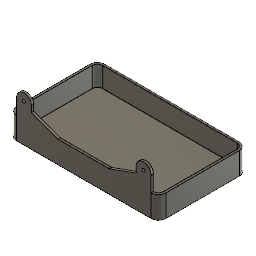
eka v1 v1 (Autodesk Fusion 360 design; units mm, degrees)
Autodesk Fusion 360 part; units mm, degrees
sketch "Sketch1" plane through (0, 0, 0) normal (0, 1, 0) x (1, 0, 0)
  line L0 (-190, 118.3432) -> (-10, 118.3432)
  line L1 (0, 108.3432) -> (0, 10)
  line L2 (-10, 0) -> (-190, 0)
  line L3 (-200, 10) -> (-200, 108.3432)
  arc A0 (-190, 118.3432) -> (-200, 108.3432) centre (-190, 108.3432) ccw
  arc A1 (-200, 10) -> (-190, 0) centre (-190, 10) ccw
  arc A2 (-10, 0) -> (0, 10) centre (-10, 10) ccw
  arc A3 (0, 108.3432) -> (-10, 118.3432) centre (-10, 108.3432) ccw
  arc A4 (-3, 108.3432) -> (-10, 115.3432) centre (-10, 108.3432) ccw
  line L4 (-190, 115.3432) -> (-10, 115.3432)
  arc A5 (-190, 115.3432) -> (-197, 108.3432) centre (-190, 108.3432) ccw
  line L5 (-197, 10) -> (-197, 108.3432)
  arc A6 (-197, 10) -> (-190, 3) centre (-190, 10) ccw
  line L6 (-10, 3) -> (-190, 3)
  arc A7 (-10, 3) -> (-3, 10) centre (-10, 10) ccw
  line L7 (-3, 108.3432) -> (-3, 10)
  dimension "d3" = 200
  dimension "d4" = 118.3432
  dimension "d6" = 10
  dimension "d7" = 10
  dimension "d8" = 10
  dimension "d9" = 10
  dimension "d15" = 3
  measures "d3" distance of L1 L3
  measures "d6" radius of A0
  measures "d7" radius of A1
  measures "d8" radius of A2
  measures "d9" radius of A3
extrude "Extrude2" add sketch "Sketch1" along normal blind 3 contours L0 L1 L2 L3 A0 A1 A2 A3 | A4 L4 A5 L5 A6 L6 A7 L7 makes body 1
extrude "Extrude3" add sketch "Sketch1" along normal blind 30 separate body makes body 2
combine "Combine1" operation add target body 2 tool bodies 1
sketch "Sketch2" plane through (0, 0, 0) normal (0, 0, 1) x (1, 0, 0)
  line L0 (-10, 0) -> (-10, 30)
  line L1 (-10, 30) -> (-190, 30)
  line L2 (-190, 30) -> (-190, 0)
  line L3 (-190, 0) -> (-10, 0)
  line L4 (-100, 30) -> (-100, 0)
  line L5 (-10, 30) -> (-10, 50)
  line L6 (-30, 50) -> (-30, 43)
  line L7 (-30, 43) -> (-65.7143, 30)
  line L8 (-10, 30) -> (-65.7143, 30)
  line L9 (-30, 50) -> (-30, 51)
  arc A0 (-10, 50) -> (-30, 51) centre (-19.975, 51) ccw
  circle A1 centre (-19.975, 51) radius 1.975
  line L10 (-170, 43) -> (-134.2857, 30)
  line L11 (-190, 30) -> (-134.2857, 30)
  line L12 (-190, 30) -> (-190, 50)
  arc A2 (-170, 51) -> (-190, 50) centre (-180.025, 51) ccw
  line L13 (-170, 50) -> (-170, 43)
  line L14 (-170, 50) -> (-170, 51)
  circle A3 centre (-180.025, 51) radius 1.975
extrude "Extrude4" add sketch "Sketch2" against normal blind 3 contours L1 L5 L6 L7 L8 L9 A0 | L1 L10 L11 L12 A2 L13 L14 bodies 2
equation "leveys = 200 mm"
equation "d3 = leveys"
equation "d4 = leveys / 1.69"
equation "fillet = 10 mm"
equation "d6 = fillet"
equation "d7 = fillet"
equation "d8 = fillet"
equation "d9 = fillet"
equation "paksuus = 30 mm"
equation "pohjanpaksuus = 3 mm"
equation "reuna = 3 mm"
equation "d15 = reuna"
equation "d16 = pohjanpaksuus"
equation "d18 = paksuus"
equation "d20 = -reuna"
